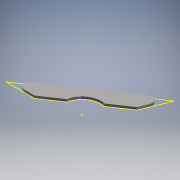
# Autodesk Inventor part: gusset
Saved by Autodesk Inventor 2018 (Build 220112000, 112)
## iProperties
Created: 2018-01-14
Part Number: gusset
Material: Stainless Steel
Document SubType Name: Modeling
Designer: prakh
Density: 8 g/cm^3
Appearance: Semi-Polished
Author: prakh
Autodesk Inventor part; units mm, degrees
ref_plane "YZ Plane" through (0, 0, 0) normal (1, 0, 0) x (0, 1, 0)
ref_plane "XZ Plane" through (0, 0, 0) normal (0, 1, 0) x (-1, 0, 0)
ref_plane "XY Plane" through (0, 0, 0) normal (0, 0, 1) x (1, 0, 0)
sketch "Sketch1" plane through (0, 0, 0) normal (0, 1, 0) x (-1, 0, 0)
  circle A0 centre (0, 0) radius 19.812
  line L0 (69.85, 0) -> (31.75, 0)
  line L1 (-12.0631, -29.3691) -> (-26.5388, -64.612)
  line L2 (-26.5388, -64.612) -> (69.85, 0)
  line L3 (69.85, 0) -> (88.796, 12.7)
  line L4 (88.796, 12.7) -> (50.696, 12.7)
  line L5 (50.696, 12.7) -> (31.75, 0)
  line L6 (-12.0631, -29.3691) -> (-31.0091, -42.0691)
  line L7 (-31.0091, -42.0691) -> (-45.4848, -77.312)
  line L8 (-45.4848, -77.312) -> (-26.5388, -64.612)
  arc A1 (-5.306, -24.8396) -> (24.9929, -4.5295) centre (0, 0) ccw
  line L9 (31.75, 0) -> (24.9929, -4.5295)
  line L10 (-5.306, -24.8396) -> (-12.0631, -29.3691)
  dimension "d0" = 112.33
  dimension "d2" = 39.624
  dimension "d3" = 31.75
  dimension "d4" = 31.75
  dimension "d5" = 38.1
  dimension "d6" = 38.1
  dimension "d7" = 112.33
  dimension "d10" = 12.7
  dimension "d12" = 12.7
  dimension "d13" = 25.4
  constraints: 22 end point, 6 collinear, 2 centre point, 2 parallel, 2 point on circle, 1 coincident, 1 concentric, 1 horizontal, 1 horizontal alignment
  measures "d0" angle of L1 L0
  measures "d2" diameter of A0
  measures "d3" distance of point (0, 0) L0.end
  measures "d4" distance of L1.start point (0, 0)
  measures "d5" distance of L1.start L1.end
  measures "d6" distance of L0.start L0.end
  measures "d10" distance between parallel lines of L7 L1
  measures "d12" distance between parallel lines of L4 L0
  measures "d13" radius of A1
extrude "Extrusion1" add sketch "Sketch1" along normal blind 3.175 contours L2 L1 L10 A1 L9 L0 | L0 L5 L4 L3 | L8 L7 L6 L1
sketch "Sketch2" plane through (0, 0, 0) normal (0, -1, 0) x (1, 0, 0)
  line L0 (45.4848, -77.312) -> (-88.796, 12.7) projected
  line L1 (31.0091, -42.0691) -> (45.4848, -77.312) projected
  line L2 (5.306, -24.8396) -> (31.0091, -42.0691) projected
  arc A0 (-24.9929, -4.5295) -> (5.306, -24.8396) centre (0, 0) ccw projected
  line L3 (-50.696, 12.7) -> (-24.9929, -4.5295) projected
  line L4 (-88.796, 12.7) -> (-50.696, 12.7) projected
fillet "Fillet1" radius 7.62 2 edges at (-88.796, 1.5875, 12.7) (45.4848, 1.5875, -77.312)
equation "\"d4\" = d3"
equation "\"d7\" = d0"
body "Solid1"
